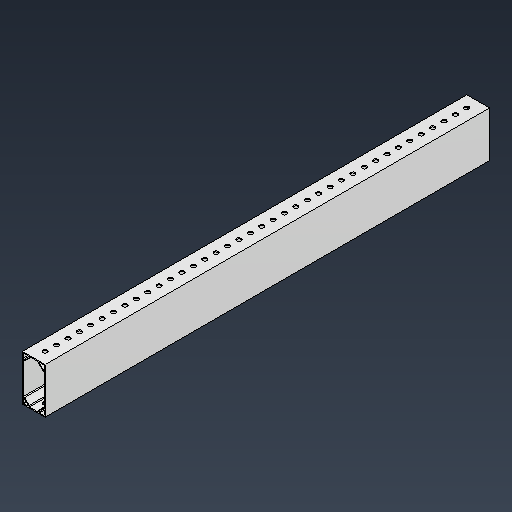
# Autodesk Inventor part: FRAME,MAXTUBE,LIGHT
Saved by Autodesk Inventor 2026 (Build 300175050, 175E)
## iProperties
Created: 2026-02-15
Part Number: FRAME,MAXTUBE,LIGHT
Material: Aluminum 6061 T6 80 Hot Formed
Document SubType Name: Modeling
Designer: Jthib
Mass: 252.257 g
Surface Area: 1780.7 cm^2
Volume: 93.4286 cm^3
Density: 2.7 g/cm^3
Appearance: Satin
Author: Jthib
Autodesk Inventor part; units mm, degrees
ref_plane "YZ Plane" through (0, 0, 0) normal (1, 0, 0) x (0, 1, 0)
ref_plane "XZ Plane" through (0, 0, 0) normal (0, 1, 0) x (-1, 0, 0)
ref_plane "XY Plane" through (0, 0, 0) normal (0, 0, 1) x (1, 0, 0)
sketch "Sketch1" plane through (0, 0, 0) normal (0, 0, 1) x (1, 0, 0)
  line L0 (12.7, -25.4) -> (-12.7, -25.4)
  line L1 (-12.7, -25.4) -> (-12.7, 25.4)
  line L2 (-12.7, 25.4) -> (12.7, 25.4)
  line L3 (12.7, 25.4) -> (12.7, -25.4)
  line L4 (12.7, -25.4) -> (-12.7, 25.4) construction
  line L5 (-12.7, -25.4) -> (12.7, 25.4) construction
  line L6 (-11.684, 23.6931) -> (-11.684, 19.3345)
  line L7 (-10.9931, 24.384) -> (-6.6345, 24.384)
  arc A0 (-6.2777, 23.1015) -> (-10.4015, 18.9777) centre (-0.015, 12.715) ccw
  arc A1 (-10.9931, 24.384) -> (-11.684, 23.6931) centre (-10.9931, 23.6931) ccw
  arc A2 (-6.2777, 23.1015) -> (-6.6345, 24.384) centre (-6.6345, 23.6931) ccw
  arc A3 (-11.684, 19.3345) -> (-10.4015, 18.9777) centre (-10.9931, 19.3345) ccw
  line L8 (-12.7, 17.6276) -> (-9.9827, 17.6276)
  arc A4 (-4.9276, 22.6827) -> (-9.9827, 17.6276) centre (-0.015, 12.715) ccw
  line L9 (-4.9276, 22.6827) -> (-4.9276, 25.4)
  line L10 (-4.9276, 24.384) -> (0, 24.384)
  line L11 (0, 35.56) -> (0, -35.56) projected
  line L12 (-17.78, 0) -> (17.78, 0) projected
  line L13 (-11.684, 17.6276) -> (-11.684, 0)
  point P0 (0, 0)
  point P1 (-11.684, 24.384)
  point P2 (0, 25.4)
  point P3 (-12.7, 0)
  dimension "d0" = 25.4
  dimension "d1" = 50.8
  dimension "d3" = 12.1285
  dimension "d4" = 1.016
  dimension "d5" = 1.016
  dimension "d6" = 0.6909
  dimension "d7" = 0.6909
  dimension "d8" = 5.7404
  dimension "d9" = 1.016
  dimension "d10" = 1.016
  dimension "d11" = 1.016
  dimension "d12" = 1.016
  constraints: 24 end point, 10 point on circle, 7 point on line, 6 perpendicular, 6 tangent, 5 centre point, 3 horizontal, 2 midpoint, 2 parallel, 1 equal radius, 1 vertical
  measures "d0" distance of L1.end L2.end
  measures "d1" distance of L0.end L1.end
  measures "d3" radius of A0
  measures "d4" distance between parallel lines of L2 L7
  measures "d5" distance between parallel lines of L1 L6
  measures "d6" radius of A1
  measures "d7" radius of A2
  measures "d9" radial gap between concentric circles of A0 A4
  measures "d10" distance edge to line of A2 L9
  measures "d11" distance between parallel lines of L2 L10
  measures "d12" distance between parallel lines of L1 L13
extrude "Extrusion1" add sketch "Sketch1" along normal blind 495.3 contours L1 L8 L13 L12 | L10 L9 L2 L11 | L1 L2 L9 A4 L8
mirror "Mirror1" about plane through (0, 0, 0) normal (1, 0, 0) of "Extrusion1"
mirror "Mirror2" about plane through (0, 0, 0) normal (0, 1, 0) of "Extrusion1", "Mirror1"
sketch "Sketch2" plane through (-12.7, 25.4, 495.3) normal (0, 1, 0) x (1, 0, 0)
  line L0 (12.7, 594.36) -> (12.7, -99.06) construction
  line L1 (-5.08, 495.3) -> (30.48, 495.3) construction
  point P0 (12.7, 495.3)
  point P1 (12.7, 482.6)
  dimension "d15" = 12.7
  constraints: 1 point on line
  measures "d15" distance from line of L1 point (12.7, 482.6)
hole "Hole1" at (0, 25.4, 12.7) direction (0, -1, 0) diameter 5.08 end through all
pattern_linear "Rectangular Pattern1" count 39 spacing 12.7 along (0, 0, 1) of "Hole1"
equation "\"d5\" = d4"
equation "\"d9\" = d4"
equation "\"d10\" = d4"
equation "\"d13\" = LENGTH"
equation "\"LENGTH\" = 495.3"
body "Solid1"
